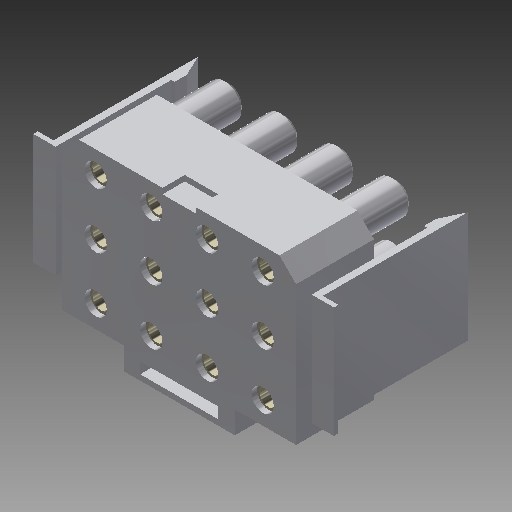
# Autodesk Inventor part: 100-13
Saved by Autodesk Inventor 2019 (Build 230136000, 136)
## iProperties
Created: 2007-12-11
Part Number: 100-13
Document SubType Name: Modeling
Designer: Autodesk Inc.
Density: 1.06 g/cm^3
Categories: <MemberInstance><Categories><Category DisplayName="" Mnemonic="CABLEANDHARNESS" InternalName="e4a7e005-5e42-4d16-b293-125e7f0d0512"><Category DisplayName="" Mnemonic="CONNECTORS" InternalName="6f634eba-a678-4820-a31d-2c2d5ee6728e"><CategoryParameter DisplayName="" Mnemonic="REFDES" InternalName="c3740e8c-60ab-4d5d-8584-52b73222f2f0"/><Category DisplayName="" Mnemonic="DISCRETEWIRE" InternalName="9a3407de-09b2-4cdb-8c40-9708d5144a28"/></Category></Category></Categories><FamilyTemplate><FamilyTemplateParameters></FamilyTemplateParameters></FamilyTemplate><CategoryParameterMap><ParamToTemplateMap><ParamToTemplate CategoryParameter="//CategoryParameter[@InternalName='c3740e8c-60ab-4d5d-8584-52b73222f2f0']" ConstantValue="PJ1"/></ParamToTemplateMap></CategoryParameterMap></MemberInstance>
Mass: 5.15771 g
Surface Area: 69.2052 cm^2
Volume: 4.86577 cm^3
Material: ABS Plastic
Description: S65 CONTROL SWITCH CONNECTOR
Appearance: Smooth - White
Company: Autodesk Inc.
GlobalPropertyList: <PropertyList/>
Component Category: Electrical
Author: Inventor
Autodesk Inventor part; units mm, degrees
ref_plane "YZ Plane" through (0, 0, 0) normal (1, 0, 0) x (0, 1, 0)
ref_plane "XZ Plane" through (0, 0, 0) normal (0, 1, 0) x (-1, 0, 0)
sketch "Sketch1" plane through (0, 0, 0) normal (0, 0, 1) x (1, 0, 0)
  line L0 (-13.335, 8.89) -> (13.335, 8.89)
  line L1 (13.335, 8.89) -> (13.335, -8.89)
  line L2 (13.335, -8.89) -> (-13.335, -8.89)
  line L3 (-13.335, -8.89) -> (-13.335, 8.89)
  circle A0 centre (-9.525, 6.35) radius 1.27
  circle A1 centre (-9.525, 6.35) radius 1.905
  line L4 (-6.35, -8.89) -> (6.35, -8.89)
  line L5 (6.35, -8.89) -> (6.35, -11.43)
  line L6 (6.35, -11.43) -> (-6.35, -11.43)
  line L7 (-6.35, -11.43) -> (-6.35, -8.89)
  line L8 (-4.445, -9.525) -> (4.445, -9.525)
  line L9 (4.445, -9.525) -> (4.445, -10.795)
  line L10 (4.445, -10.795) -> (-4.445, -10.795)
  line L11 (-4.445, -10.795) -> (-4.445, -9.525)
  point P0 (0, 0)
  point P1 (-13.335, 0)
  point P2 (0, 8.89)
  point P3 (0, -10.795)
  point P4 (0, -11.43)
  point P5 (0, -9.525)
  dimension "Length" = 26.67
  dimension "Width" = 17.78
  dimension "Hole_Dia" = 2.54
  dimension "Hole_Shell_Dia" = 3.81
  dimension "Origin_Hole_Y" = 2.54
  dimension "Origin_Hole_X" = 3.81
  dimension "d18" = 1.27
  dimension "Tab_Space_Y" = 0.635
  dimension "d20" = 0.635
  dimension "Tab_Space_X" = 1.905
  dimension "Bot_Tab_Length" = 12.7
  constraints: 24 end point, 6 parallel, 5 midpoint, 3 horizontal, 3 perpendicular, 3 vertical alignment, 2 centre point, 1 coincident, 1 horizontal alignment, 1 point on line
  measures "Length" distance of L0.start L0.end
  measures "Width" distance of L2.end L0.start
  measures "Hole_Dia" diameter of A0
  measures "Hole_Shell_Dia" diameter of A1
  measures "Origin_Hole_Y" distance from line of L0 A0.centre
  measures "Origin_Hole_X" distance from line of L3 A0.centre
  measures "d18" distance of L8.end L9.end
  measures "Tab_Space_Y" distance between parallel lines of L4 L8
  measures "d20" distance between parallel lines of L6 L10
  measures "Tab_Space_X" distance between parallel lines of L7 L11
  measures "Bot_Tab_Length" distance of L5.end L6.end
extrude "Extrusion1" add sketch "Sketch1" along normal blind 8.89 contours L0 L1 L2 L3 | L2 L5 L6 L7 | A0 | A1
extrude "Extrusion2" add sketch "Sketch1" against normal blind 6.35 contours A1
extrude "Extrusion3" cut sketch "Sketch1" along normal up to next contours A0
pattern_linear "Rectangular Pattern1" count 4 spacing 6.35 along (1, 0, 0) count 3 spacing 6.35 along (0, -1, 0) of "Extrusion2", "Extrusion3"
chamfer "Chamfer1" distance 1.905 angle 45 2 edges at (-13.335, 8.89, 4.445) (13.335, 8.89, 4.445)
sketch "Sketch2" plane through (0, 0, 8.89) normal (0, 0, 1) x (1, 0, 0)
  line L0 (-1.905, 8.89) -> (1.905, 8.89)
  line L1 (1.905, 8.89) -> (1.905, 8.255)
  line L2 (1.905, 8.255) -> (-1.905, 8.255)
  line L3 (-1.905, 8.255) -> (-1.905, 8.89)
  line L4 (-11.43, 8.89) -> (11.43, 8.89) projected
  point P0 (0, 0)
  point P1 (0, 8.255)
  dimension "d26" = 3.81
  dimension "d27" = 0.635
  constraints: 8 end point, 2 parallel, 1 collinear, 1 horizontal, 1 midpoint, 1 perpendicular, 1 vertical alignment
  measures "d26" distance of L1.end L2.end
  measures "d27" distance between parallel lines of L0 L2
extrude "Extrusion4" cut sketch "Sketch2" against normal blind 2.54
sketch "Sketch3" plane through (0, 0, 0) normal (0, 1, 0) x (-1, 0, 0)
  line L0 (13.335, 0) -> (13.335, 8.89) projected
  line L1 (13.335, 3.175) -> (14.605, 3.175)
  line L2 (14.605, 3.175) -> (14.605, 5.715)
  line L3 (14.605, 5.715) -> (13.335, 5.715)
  line L4 (13.335, 5.715) -> (13.335, 3.175)
  line L5 (14.605, 3.175) -> (14.605, -4.826)
  line L6 (14.605, -4.826) -> (14.224, -4.826)
  line L7 (14.224, -4.826) -> (14.224, -6.1848)
  line L8 (14.224, -6.1848) -> (15.367, -8.636)
  line L9 (15.367, -8.636) -> (15.367, 7.874)
  line L10 (15.367, 7.874) -> (17.145, 7.874)
  line L11 (17.145, 7.874) -> (17.145, 8.382)
  line L12 (17.145, 8.382) -> (14.605, 8.382)
  line L13 (14.605, 5.715) -> (14.605, 8.382)
  line L14 (6.35, 8.89) -> (13.335, 8.89) projected
  point P0 (0, 0)
  point P1 (13.335, 4.445)
  point P2 (13.335, 4.445)
  dimension "d30" = 1.27
  dimension "d31" = 2.54
  dimension "d32" = 0.508
  dimension "d34" = 0.508
  dimension "d35" = 2.54
  dimension "d36" = 0.762
  dimension "d37" = 0.381
  dimension "d38" = 25
  dimension "d39" = 16.51
  dimension "d40" = 3.81
  constraints: 26 end point, 8 parallel, 3 perpendicular, 2 midpoint, 1 coincident, 1 horizontal, 1 point on line
  measures "d30" distance of L1.start L1.end
  measures "d31" distance of L1.end L2.end
  measures "d32" distance between parallel lines of L12 L14
  measures "d34" distance between parallel lines of L10 L12
  measures "d35" distance between parallel lines of L13 L11
  measures "d36" distance between parallel lines of L13 L9
  measures "d37" distance of L5.end L6.end
  measures "d38" angle of L9 L8
  measures "d39" distance of L8.end L9.end
  measures "d40" distance from line of L8.end L6
extrude "Extrusion5" add sketch "Sketch3" along normal mid plane 1.905 contours L0 L3 L2 L1
extrude "Extrusion6" add sketch "Sketch3" along normal mid plane 12.7 contours L2 L13 L12 L11 L10 L9 L8 L7 L6 L5
mirror "Mirror1" about plane through (0, 0, 0) normal (1, 0, 0) of "Extrusion6", "Extrusion5"
chamfer "Chamfer2" distance 0.508 angle 45 12 edges at (7.62, 6.35, -6.35) (1.27, 6.35, -6.35) (-5.08, 6.35, -6.35) (-11.43, 6.35, -6.35) (-11.43, 0, -6.35) (-5.08, 0, -6.35) (1.27, 0, -6.35) (7.62, 0, -6.35) (7.62, -6.35, -6.35) (1.27, -6.35, -6.35) (-5.08, -6.35, -6.35) (-11.43, -6.35, -6.35)
ref_plane "Work Plane1" through (-9.525, 6.35, 0) normal (-1, 0, 0) x (0, 0, 1)
sketch "Sketch4" plane through (-9.525, 6.35, 0) normal (-1, 0, 0) x (0, 0, 1)
  line L0 (-9.398, 0) -> (11.938, 0) projected
  arc A0 (-5.0979, 0) -> (-4.4629, -0.635) centre (-4.4629, 0) ccw
  line L1 (1.2521, -0.635) -> (-4.4629, -0.635)
  line L2 (-5.0979, 0) -> (1.2521, 0)
  line L3 (-6.35, -1.27) -> (8.89, -1.27) projected
  line L4 (1.2521, -0.635) -> (2.159, -1.27)
  line L5 (8.255, -1.27) -> (8.255, -1.016)
  line L6 (8.89, 1.27) -> (8.89, -1.27) projected
  line L7 (1.2521, 0) -> (8.255, 0)
  arc A1 (-4.8439, 0) -> (-4.4629, -0.381) centre (-4.4629, 0) ccw
  line L8 (-4.4629, -0.381) -> (1.3322, -0.381)
  line L9 (1.3322, -0.381) -> (2.2391, -1.016)
  line L10 (2.2391, -1.016) -> (8.255, -1.016)
  point P0 (0, -6.35)
  dimension "d49" = 1.27
  dimension "d51" = 145
  dimension "d53" = 6.096
  dimension "d54" = 0.635
  dimension "d55" = 5.715
  dimension "d56" = 0.254
  dimension "d57" = 0.254
  dimension "d58" = 0.254
  constraints: 16 end point, 6 point on line, 4 point on circle, 2 centre point, 2 horizontal, 1 collinear, 1 parallel, 1 perpendicular, 1 tangent, 1 other
  measures "d49" diameter of A0
  measures "d51" angle of L1 L4
  measures "d53" distance from line of L5 L4.end
  measures "d54" distance between parallel lines of L5 L6
  measures "d55" horizontal distance of A0.centre L1.start
  measures "d56" distance between parallel lines of L10 L3
  measures "d57" distance between parallel lines of L4 L9
  measures "d58" radial gap between concentric circles of A0 A1
revolve "Revolution1" add sketch "Sketch4" angle 360 about axis through (-9.525, 6.35, 0) along (0, 0, 1) separate body contours L0 A1 L8 L9 L10 L5 L3 L4 L1 A0
pattern_linear "Rectangular Pattern2" count 4 spacing 6.35 along (1, 0, 0) count 3 spacing 6.35 along (0, -1, 0) of "Revolution1" bodies 2
equation "\"d20\" = Tab_Space_Y"
equation "\"d34\" = d32"
equation "\"d57\" = d56"
equation "\"d62\" = Occurence_Space_X"
equation "\"d65\" = Occurence_Space_Y"
equation "\"Occurence_Space_X\" = 6.35"
equation "\"Occurence_Space_Y\" = 6.35"
body "Solid1"
body "Solid2"
